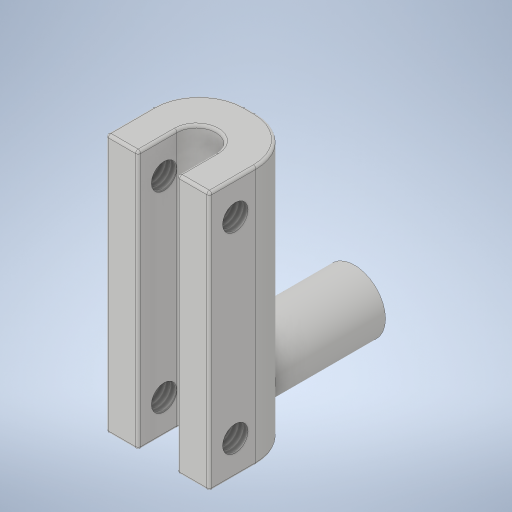
# Autodesk Inventor part: StepperToSpout_Gerion_V3
Saved by Autodesk Inventor 2023 (Build 270158000, 158)
## iProperties
Created: 2019-09-20
Part Number: StepperToSpout_Gerion_V3
Material: Generic
Document SubType Name: Modeling
Designer: Xiaonan Richard Sun
Density: 1 g/cm^3
Appearance: Default
Author: Xiaonan Richard Sun
Autodesk Inventor part; units mm, degrees
ref_plane "YZ Plane" through (0, 0, 0) normal (1, 0, 0) x (0, 1, 0)
ref_plane "XZ Plane" through (0, 0, 0) normal (0, 1, 0) x (-1, 0, 0)
ref_plane "XY Plane" through (0, 0, 0) normal (0, 0, 1) x (1, 0, 0)
sketch "Sketch1" plane through (0, 0, 0) normal (0, 0, 1) x (1, 0, 0)
  line L0 (0, 0) -> (10, 0)
  line L1 (10, 0) -> (10, 25)
  line L2 (10, 25) -> (0, 25)
  line L3 (0, 25) -> (0, 0)
  dimension "d0" = 10
  dimension "d1" = 25
  constraints: 8 end point, 2 parallel, 1 horizontal, 1 perpendicular
  measures "d0" distance of L2.end L1.end
  measures "d1" distance of L1.end L0.end
extrude "Extrusion1" add sketch "Sketch1" along normal blind 9
sketch "Sketch2" plane through (0, 0, 0) normal (0, 0, -1) x (-1, 0, 0)
  arc A0 (-3.4183, 2.63) -> (-6.5817, 2.63) centre (-5, 4) ccw
  arc A1 (-3.4183, 2.63) -> (-6.5817, 2.63) centre (-5, 4) ccw
  circle A2 centre (-5, 4) radius 3
  line L0 (0, 25) -> (0, 0) construction
  line L1 (0, 0) -> (-10, 0) construction
  line L2 (-6.5817, 2.63) -> (-3.4183, 2.63)
  line L3 (-5, 0) -> (-5, 25) construction
  line L4 (-10, 25) -> (0, 25) construction
  dimension "d7" = 4.185
  dimension "d9" = 6
  dimension "d35" = 3.1633
  dimension "d50" = 4
  constraints: 4 end point, 4 point on circle, 3 centre point, 2 midpoint, 1 coincident, 1 concentric, 1 horizontal, 1 point on line
  measures "d7" diameter of A0
  measures "d9" diameter of A2
  measures "d35" distance of L2.start L2.end
  measures "d50" distance from line of L1 A0.centre
extrude "Extrusion2" add sketch "Sketch2" along normal blind 10
sketch "Sketch4" plane through (0, 25, 0) normal (0, 1, 0) x (1, 0, 0)
  arc A0 (6.875, -5.25) -> (3.125, -5.25) centre (5, -5.25) ccw
  line L0 (3.125, -5.25) -> (3.125, -9)
  line L1 (6.875, -9) -> (6.875, -5.25)
  line L2 (10, -9) -> (0, -9) construction
  line L3 (6.875, -9) -> (3.125, -9)
  line L4 (10, 0) -> (0, 0) construction
  line L5 (5, 0) -> (5, -9) construction
  dimension "d14" = 3.75
  dimension "d39" = 3.75
  dimension "d53" = 3.75
  constraints: 8 end point, 3 point on line, 2 midpoint, 2 point on circle, 2 tangent, 1 centre point, 1 collinear, 1 perpendicular, 1 vertical
  measures "d14" diameter of A0
  measures "d39" distance between parallel lines of L0 L1
  measures "d53" distance from line of A0.centre L2
extrude "Extrusion4" cut sketch "Sketch4" against normal blind 25
sketch "Sketch8" plane through (0, 0, 9) normal (0, 0, 1) x (1, 0, 0)
  line L0 (2.3, 19) -> (7.7, 19)
  line L1 (7.7, 19) -> (7.7, 6)
  line L2 (7.7, 6) -> (2.3, 6)
  line L3 (2.3, 6) -> (2.3, 19)
  line L4 (6.875, 25) -> (6.875, 0) construction
  line L5 (6.875, 0) -> (10, 0) construction
  line L6 (10, 0) -> (10, 25) construction
  line L7 (10, 25) -> (6.875, 25) construction
  line L8 (3.125, 0) -> (3.125, 25) construction
  line L9 (3.125, 25) -> (0, 25) construction
  line L10 (0, 25) -> (0, 0) construction
  line L11 (0, 0) -> (3.125, 0) construction
  dimension "d54" = 6
  dimension "d55" = 6
  dimension "d56" = 2.3
  dimension "d57" = 2.3
  constraints: 8 end point, 2 parallel, 1 horizontal, 1 perpendicular
  measures "d54" distance between parallel lines of L5 L2
  measures "d55" distance between parallel lines of L7 L0
  measures "d56" distance between parallel lines of L6 L1
  measures "d57" distance between parallel lines of L10 L3
extrude "Extrusion6" [suppressed]
sketch "Sketch6" plane through (0, 6.7085, 2.6824) normal (-1, 0, 0) x (0, 0, 1)
  line L0 (-2.6824, 18.2915) -> (6.3176, 18.2915) construction
  line L1 (6.3176, 18.2915) -> (6.3176, -6.7085) construction
  line L2 (-2.6824, -6.7085) -> (6.3176, -6.7085) construction
  point P0 (3.8176, 15.0415)
  point P1 (3.8176, -3.4585)
  dimension "d47" = 3.25
  dimension "d58" = 2.5
  dimension "d59" = 3.25
  dimension "d60" = 2.5
  measures "d47" distance from line of point (3.818, 15.042) L0
  measures "d58" distance from line of L1 point (3.818, 15.042)
  measures "d59" distance from line of L2 point (3.818, -3.458)
  measures "d60" distance from line of L1 point (3.818, -3.458)
hole "Hole1" at (0, 21.75, 6.5) at (0, 3.25, 6.5) direction (1, 0, 0) diameter 2.459 end through all thread size "M3x0.5" class "6H" standard "ISO Metric profile"
fillet "Fillet2" radius 4.5 2 edges at (10, 12.5, 0) (0, 12.5, 0)
fillet "Fillet2" radius 0.25 21 edges at (10, 12.5, 9) (6.875, 12.5, 9) (3.125, 12.5, 9) (0, 12.5, 9) (1.5625, 25, 9) (1.5625, 0, 9) (5, 25, 3.375) (6.875, 25, 7.125) (3.125, 25, 7.125) (5, 0, 3.375) (6.875, 0, 7.125) (3.125, 0, 7.125) (8.4375, 25, 9) (8.4375, 0, 9) (10, 25, 4.5) (10, 0, 4.5) (5, 25, 0) (5, 0, 0) (0, 0, 4.5) (0, 25, 4.5) (8, 4, 0)
sketch "Sketch9" plane through (5, 4, -10) normal (0, 0, -1) x (-1, 0, 0)
  arc A0 (1.5817, -1.37) -> (-1.5817, -1.37) centre (0, 0) ccw construction
  arc A1 (0.4615, 2.9643) -> (-0.4615, 2.9643) centre (0, 0) ccw construction
  circle A2 centre (0, 0) radius 2.0925
  point P0 (5, -4)
  point P1 (-2.7692, 1.1538)
  point P2 (2.7692, 1.1538)
  constraints: 1 centre point, 1 coincident, 1 concentric
extrude "Extrusion7" cut sketch "Sketch9" against normal up to surface (10 mm away)
sketch "Sketch10" plane through (0, 0, 0) normal (0, 0, -1) x (-1, 0, 0)
  line L0 (-3, 16) -> (-3, 8) construction
  line L1 (-3, 8) -> (-7, 8) construction
  line L2 (-7, 8) -> (-7, 16) construction
  line L3 (-7, 16) -> (-3, 16) construction
  arc A0 (-4.5, 7.2113) -> (-5.5, 7.2113) centre (-5, 4) ccw construction
  line L4 (-5, 7.25) -> (-5, 25) construction
  line L5 (-4.5, 25) -> (-5.5, 25) construction
  line L6 (-3.5491, 14.0041) -> (-4.5491, 14.3485)
  line L7 (-4.5491, 14.3485) -> (-4.5491, 14.4919)
  line L8 (-4.5491, 14.4919) -> (-3.5491, 14.8363)
  line L9 (-3.5491, 14.8363) -> (-3.5491, 14.6937)
  line L10 (-3.5491, 14.6937) -> (-4.3798, 14.4165)
  line L11 (-4.3798, 14.4165) -> (-3.5491, 14.1394)
  line L12 (-3.5491, 14.1394) -> (-3.5491, 14.0041)
  spline S0 degree 2 poles (-4.5661, 13.5924) (-4.5661, 13.7723) (-4.3644, 13.97) (-4.178, 13.97) knots 0 0 0 1 2 2 2
  spline S1 degree 2 poles (-4.178, 13.97) (-3.9948, 13.97) (-3.7777, 13.778) (-3.7777, 13.6232) knots 0 0 0 1 2 2 2
  spline S2 degree 2 poles (-3.7777, 13.6232) (-3.7777, 13.5535) (-3.8182, 13.4457) (-3.8611, 13.406) knots 0 0 0 1 2 2 2
  spline S3 degree 2 poles (-3.8611, 13.406) (-3.9041, 13.3655) (-4.0281, 13.3225) (-4.118, 13.3225) knots 0 0 0 1 2 2 2
  line L13 (-4.118, 13.3225) -> (-4.1869, 13.3225)
  line L14 (-4.1869, 13.3225) -> (-4.1869, 13.842)
  spline S4 degree 2 poles (-4.1869, 13.842) (-4.3174, 13.842) (-4.4559, 13.7107) (-4.4559, 13.594) knots 0 0 0 1 2 2 2
  spline S5 degree 2 poles (-4.4559, 13.594) (-4.4559, 13.5527) (-4.4373, 13.4724) (-4.4227, 13.44) knots 0 0 0 1 2 2 2
  spline S6 degree 2 poles (-4.4227, 13.44) (-4.4065, 13.406) (-4.3781, 13.359) (-4.3652, 13.3436) knots 0 0 0 1 2 2 2
  line L15 (-4.3652, 13.3436) -> (-4.3652, 13.3363)
  line L16 (-4.3652, 13.3363) -> (-4.5029, 13.3363)
  spline S7 degree 2 poles (-4.5029, 13.3363) (-4.5119, 13.3582) (-4.5378, 13.4246) (-4.5451, 13.4506) knots 0 0 0 1 2 2 2
  spline S8 degree 2 poles (-4.5451, 13.4506) (-4.5556, 13.487) (-4.5661, 13.547) (-4.5661, 13.5924) knots 0 0 0 1 2 2 2
  spline S9 degree 2 poles (-4.0905, 13.4457) (-4.0394, 13.4473) (-3.9649, 13.4684) (-3.9397, 13.4887) knots 0 0 0 1 2 2 2
  spline S10 degree 2 poles (-3.9397, 13.4887) (-3.9114, 13.5105) (-3.8814, 13.5794) (-3.8814, 13.6305) knots 0 0 0 1 2 2 2
  spline S11 degree 2 poles (-3.8814, 13.6305) (-3.8814, 13.6807) (-3.9114, 13.7512) (-3.9405, 13.7804) knots 0 0 0 1 2 2 2
  spline S12 degree 2 poles (-3.9405, 13.7804) (-3.9705, 13.8088) (-4.0426, 13.8379) (-4.0905, 13.842) knots 0 0 0 1 2 2 2
  line L17 (-4.0905, 13.842) -> (-4.0905, 13.4457)
  line L18 (-3.9341, 12.7966) -> (-3.9341, 12.8031)
  spline S13 degree 2 poles (-3.9341, 12.8031) (-3.93, 12.8177) (-3.9284, 12.8493) (-3.9284, 12.8712) knots 0 0 0 1 2 2 2
  spline S14 degree 2 poles (-3.9284, 12.8712) (-3.9284, 12.9222) (-3.973, 13.0227) (-4.0167, 13.0681) knots 0 0 0 1 2 2 2
  line L19 (-4.0167, 13.0681) -> (-4.5491, 13.0681)
  line L20 (-4.5491, 13.0681) -> (-4.5491, 13.1945)
  line L21 (-4.5491, 13.1945) -> (-3.7987, 13.1945)
  line L22 (-3.7987, 13.1945) -> (-3.7987, 13.0681)
  line L23 (-3.7987, 13.0681) -> (-3.9106, 13.0681)
  spline S15 degree 2 poles (-3.9106, 13.0681) (-3.849, 12.9992) (-3.7987, 12.8963) (-3.7987, 12.8477) knots 0 0 0 1 2 2 2
  spline S16 degree 2 poles (-3.7987, 12.8477) (-3.7987, 12.8282) (-3.8003, 12.8088) (-3.8028, 12.7966) knots 0 0 0 1 2 2 2
  line L24 (-3.8028, 12.7966) -> (-3.9341, 12.7966)
  spline S17 degree 2 poles (-4.567, 12.4959) (-4.567, 12.5713) (-4.5264, 12.7018) (-4.5037, 12.7447) knots 0 0 0 1 2 2 2
  line L25 (-4.5037, 12.7447) -> (-4.3619, 12.7447)
  line L26 (-4.3619, 12.7447) -> (-4.3619, 12.7382)
  spline S18 degree 2 poles (-4.3619, 12.7382) (-4.3749, 12.722) (-4.4057, 12.6783) (-4.4227, 12.6418) knots 0 0 0 1 2 2 2
  spline S19 degree 2 poles (-4.4227, 12.6418) (-4.4381, 12.6102) (-4.4608, 12.5324) (-4.4608, 12.4911) knots 0 0 0 1 2 2 2
  spline S20 degree 2 poles (-4.4608, 12.4911) (-4.4608, 12.4611) (-4.447, 12.3922) (-4.4357, 12.376) knots 0 0 0 1 2 2 2
  spline S21 degree 2 poles (-4.4357, 12.376) (-4.4203, 12.3525) (-4.3854, 12.3314) (-4.3498, 12.3314) knots 0 0 0 1 2 2 2
  spline S22 degree 2 poles (-4.3498, 12.3314) (-4.3052, 12.3314) (-4.259, 12.3801) (-4.2436, 12.4425) knots 0 0 0 1 2 2 2
  spline S23 degree 2 poles (-4.2436, 12.4425) (-4.2379, 12.4668) (-4.2217, 12.5446) (-4.2128, 12.5778) knots 0 0 0 1 2 2 2
  spline S24 degree 2 poles (-4.2128, 12.5778) (-4.1877, 12.6637) (-4.084, 12.7415) (-4.0102, 12.7415) knots 0 0 0 1 2 2 2
  spline S25 degree 2 poles (-4.0102, 12.7415) (-3.9081, 12.7415) (-3.7809, 12.5883) (-3.7809, 12.4619) knots 0 0 0 1 2 2 2
  spline S26 degree 2 poles (-3.7809, 12.4619) (-3.7809, 12.3995) (-3.8117, 12.2731) (-3.8352, 12.2301) knots 0 0 0 1 2 2 2
  line L27 (-3.8352, 12.2301) -> (-3.9705, 12.2301)
  line L28 (-3.9705, 12.2301) -> (-3.9705, 12.2366)
  spline S27 degree 2 poles (-3.9705, 12.2366) (-3.9316, 12.2853) (-3.8871, 12.4036) (-3.8871, 12.4643) knots 0 0 0 1 2 2 2
  spline S28 degree 2 poles (-3.8871, 12.4643) (-3.8871, 12.5267) (-3.9397, 12.6126) (-3.9924, 12.6126) knots 0 0 0 1 2 2 2
  spline S29 degree 2 poles (-3.9924, 12.6126) (-4.0402, 12.6126) (-4.0864, 12.5616) (-4.101, 12.5049) knots 0 0 0 1 2 2 2
  spline S30 degree 2 poles (-4.101, 12.5049) (-4.1083, 12.4773) (-4.1229, 12.4076) (-4.1318, 12.3695) knots 0 0 0 1 2 2 2
  spline S31 degree 2 poles (-4.1318, 12.3695) (-4.1529, 12.2869) (-4.2493, 12.2026) (-4.3328, 12.2026) knots 0 0 0 1 2 2 2
  spline S32 degree 2 poles (-4.3328, 12.2026) (-4.3814, 12.2026) (-4.4673, 12.2407) (-4.4989, 12.278) knots 0 0 0 1 2 2 2
  spline S33 degree 2 poles (-4.4989, 12.278) (-4.5321, 12.3177) (-4.567, 12.419) (-4.567, 12.4959) knots 0 0 0 1 2 2 2
  line L29 (-4.5491, 11.9562) -> (-4.5491, 12.0827)
  line L30 (-4.5491, 12.0827) -> (-3.7987, 12.0827)
  line L31 (-3.7987, 12.0827) -> (-3.7987, 11.9562)
  line L32 (-3.7987, 11.9562) -> (-4.5491, 11.9562)
  line L33 (-3.6739, 11.9473) -> (-3.6739, 12.0908)
  line L34 (-3.6739, 12.0908) -> (-3.5426, 12.0908)
  line L35 (-3.5426, 12.0908) -> (-3.5426, 11.9473)
  line L36 (-3.5426, 11.9473) -> (-3.6739, 11.9473)
  spline S34 degree 2 poles (-4.1739, 11.154) (-4.3636, 11.154) (-4.5702, 11.3363) (-4.5702, 11.4887) knots 0 0 0 1 2 2 2
  spline S35 degree 2 poles (-4.5702, 11.4887) (-4.5702, 11.6451) (-4.3571, 11.8241) (-4.1739, 11.8241) knots 0 0 0 1 2 2 2
  spline S36 degree 2 poles (-4.1739, 11.8241) (-3.9859, 11.8241) (-3.7777, 11.6394) (-3.7777, 11.4887) knots 0 0 0 1 2 2 2
  spline S37 degree 2 poles (-3.7777, 11.4887) (-3.7777, 11.3363) (-3.9851, 11.154) (-4.1739, 11.154) knots 0 0 0 1 2 2 2
  spline S38 degree 2 poles (-4.1739, 11.2844) (-4.0281, 11.2844) (-3.8862, 11.3906) (-3.8862, 11.4887) knots 0 0 0 1 2 2 2
  spline S39 degree 2 poles (-3.8862, 11.4887) (-3.8862, 11.5867) (-4.0281, 11.6937) (-4.1739, 11.6937) knots 0 0 0 1 2 2 2
  spline S40 degree 2 poles (-4.1739, 11.6937) (-4.3157, 11.6937) (-4.4616, 11.5867) (-4.4616, 11.4887) knots 0 0 0 1 2 2 2
  spline S41 degree 2 poles (-4.4616, 11.4887) (-4.4616, 11.3914) (-4.3182, 11.2844) (-4.1739, 11.2844) knots 0 0 0 1 2 2 2
  line L37 (-4.5491, 10.4352) -> (-4.5491, 10.5616)
  line L38 (-4.5491, 10.5616) -> (-4.1213, 10.5616)
  spline S42 degree 2 poles (-4.1213, 10.5616) (-4.0694, 10.5616) (-3.9802, 10.5713) (-3.9535, 10.5859) knots 0 0 0 1 2 2 2
  spline S43 degree 2 poles (-3.9535, 10.5859) (-3.9251, 10.6013) (-3.8976, 10.6564) (-3.8976, 10.7034) knots 0 0 0 1 2 2 2
  spline S44 degree 2 poles (-3.8976, 10.7034) (-3.8976, 10.7504) (-3.9478, 10.8501) (-3.9884, 10.8979) knots 0 0 0 1 2 2 2
  line L39 (-3.9884, 10.8979) -> (-4.5491, 10.8979)
  line L40 (-4.5491, 10.8979) -> (-4.5491, 11.0243)
  line L41 (-4.5491, 11.0243) -> (-3.7987, 11.0243)
  line L42 (-3.7987, 11.0243) -> (-3.7987, 10.8979)
  line L43 (-3.7987, 10.8979) -> (-3.8822, 10.8979)
  spline S45 degree 2 poles (-3.8822, 10.8979) (-3.8311, 10.8412) (-3.7777, 10.7318) (-3.7777, 10.6702) knots 0 0 0 1 2 2 2
  spline S46 degree 2 poles (-3.7777, 10.6702) (-3.7777, 10.56) (-3.9235, 10.4352) (-4.0621, 10.4352) knots 0 0 0 1 2 2 2
  line L44 (-4.0621, 10.4352) -> (-4.5491, 10.4352)
  spline S47 degree 2 poles (-3.6439, 9.577) (-3.6439, 9.6135) (-3.6618, 9.6856) (-3.6755, 9.7204) knots 0 0 0 1 2 2 2
  spline S48 degree 2 poles (-3.6755, 9.7204) (-3.6893, 9.7528) (-3.7185, 9.8006) (-3.7315, 9.8193) knots 0 0 0 1 2 2 2
  line L45 (-3.7315, 9.8193) -> (-3.7315, 9.8274)
  line L46 (-3.7315, 9.8274) -> (-3.5896, 9.8274)
  spline S49 degree 2 poles (-3.5896, 9.8274) (-3.5661, 9.7836) (-3.5281, 9.6337) (-3.5281, 9.5665) knots 0 0 0 1 2 2 2
  spline S50 degree 2 poles (-3.5281, 9.5665) (-3.5281, 9.4984) (-3.5556, 9.3971) (-3.5848, 9.3558) knots 0 0 0 1 2 2 2
  spline S51 degree 2 poles (-3.5848, 9.3558) (-3.6164, 9.312) (-3.708, 9.2666) (-3.7696, 9.2666) knots 0 0 0 1 2 2 2
  spline S52 degree 2 poles (-3.7696, 9.2666) (-3.8522, 9.2666) (-3.977, 9.3752) (-3.9932, 9.4514) knots 0 0 0 1 2 2 2
  line L47 (-3.9932, 9.4514) -> (-4.0029, 9.4514)
  spline S53 degree 2 poles (-4.0029, 9.4514) (-4.0094, 9.4198) (-4.0386, 9.3477) (-4.0678, 9.3169) knots 0 0 0 1 2 2 2
  spline S54 degree 2 poles (-4.0678, 9.3169) (-4.0961, 9.2861) (-4.1869, 9.2472) (-4.2525, 9.2472) knots 0 0 0 1 2 2 2
  spline S55 degree 2 poles (-4.2525, 9.2472) (-4.3198, 9.2472) (-4.4341, 9.2934) (-4.4778, 9.3355) knots 0 0 0 1 2 2 2
  spline S56 degree 2 poles (-4.4778, 9.3355) (-4.5232, 9.3793) (-4.5702, 9.5032) (-4.5702, 9.5818) knots 0 0 0 1 2 2 2
  spline S57 degree 2 poles (-4.5702, 9.5818) (-4.5702, 9.6572) (-4.5337, 9.8047) (-4.5086, 9.8549) knots 0 0 0 1 2 2 2
  line L48 (-4.5086, 9.8549) -> (-4.3668, 9.8549)
  line L49 (-4.3668, 9.8549) -> (-4.3668, 9.8452)
  spline S58 degree 2 poles (-4.3668, 9.8452) (-4.3976, 9.8031) (-4.4543, 9.6605) (-4.4543, 9.59) knots 0 0 0 1 2 2 2
  spline S59 degree 2 poles (-4.4543, 9.59) (-4.4543, 9.5486) (-4.4284, 9.466) (-4.3984, 9.4384) knots 0 0 0 1 2 2 2
  spline S60 degree 2 poles (-4.3984, 9.4384) (-4.3684, 9.4117) (-4.2971, 9.3833) (-4.2428, 9.3833) knots 0 0 0 1 2 2 2
  spline S61 degree 2 poles (-4.2428, 9.3833) (-4.1885, 9.3833) (-4.118, 9.4149) (-4.0978, 9.4433) knots 0 0 0 1 2 2 2
  spline S62 degree 2 poles (-4.0978, 9.4433) (-4.0775, 9.4716) (-4.0621, 9.5486) (-4.0621, 9.594) knots 0 0 0 1 2 2 2
  line L50 (-4.0621, 9.594) -> (-4.0621, 9.6507)
  line L51 (-4.0621, 9.6507) -> (-3.9511, 9.6507)
  line L52 (-3.9511, 9.6507) -> (-3.9511, 9.6062)
  spline S63 degree 2 poles (-3.9511, 9.6062) (-3.9511, 9.5162) (-3.8652, 9.4028) (-3.7833, 9.4028) knots 0 0 0 1 2 2 2
  spline S64 degree 2 poles (-3.7833, 9.4028) (-3.7452, 9.4028) (-3.6909, 9.4319) (-3.6747, 9.4554) knots 0 0 0 1 2 2 2
  spline S65 degree 2 poles (-3.6747, 9.4554) (-3.6577, 9.4806) (-3.6439, 9.5421) (-3.6439, 9.577) knots 0 0 0 1 2 2 2
  spline S66 degree 2 poles (-5.8885, 14.1653) (-5.963, 14.1653) (-6.0773, 14.222) (-6.1146, 14.269) knots 0 0 0 1 2 2 2
  spline S67 degree 2 poles (-6.1146, 14.269) (-6.1583, 14.3258) (-6.1956, 14.4546) (-6.1956, 14.5567) knots 0 0 0 1 2 2 2
  line L53 (-6.1956, 14.5567) -> (-6.1956, 14.8436)
  line L54 (-6.1956, 14.8436) -> (-5.1956, 14.8436)
  line L55 (-5.1956, 14.8436) -> (-5.1956, 14.5786)
  spline S68 degree 2 poles (-5.1956, 14.5786) (-5.1956, 14.4716) (-5.2094, 14.3647) (-5.2361, 14.316) knots 0 0 0 1 2 2 2
  spline S69 degree 2 poles (-5.2361, 14.316) (-5.2645, 14.2618) (-5.3577, 14.2123) (-5.4209, 14.2123) knots 0 0 0 1 2 2 2
  spline S70 degree 2 poles (-5.4209, 14.2123) (-5.4914, 14.2123) (-5.6032, 14.2869) (-5.6348, 14.3525) knots 0 0 0 1 2 2 2
  line L56 (-5.6348, 14.3525) -> (-5.6397, 14.3525)
  spline S71 degree 2 poles (-5.6397, 14.3525) (-5.664, 14.2634) (-5.7928, 14.1653) (-5.8885, 14.1653) knots 0 0 0 1 2 2 2
  spline S72 degree 2 poles (-5.8941, 14.3039) (-5.8374, 14.3039) (-5.7645, 14.3363) (-5.7386, 14.3849) knots 0 0 0 1 2 2 2
  spline S73 degree 2 poles (-5.7386, 14.3849) (-5.7223, 14.4165) (-5.7126, 14.4911) (-5.7126, 14.56) knots 0 0 0 1 2 2 2
  line L57 (-5.7126, 14.56) -> (-5.7126, 14.7107)
  line L58 (-5.7126, 14.7107) -> (-6.0822, 14.7107)
  line L59 (-6.0822, 14.7107) -> (-6.0822, 14.6029)
  spline S74 degree 2 poles (-6.0822, 14.6029) (-6.0822, 14.5154) (-6.0659, 14.4149) (-6.04, 14.376) knots 0 0 0 1 2 2 2
  spline S75 degree 2 poles (-6.04, 14.376) (-6.0133, 14.3387) (-5.9468, 14.3039) (-5.8941, 14.3039) knots 0 0 0 1 2 2 2
  spline S76 degree 2 poles (-5.4395, 14.3509) (-5.4039, 14.3509) (-5.3504, 14.3752) (-5.335, 14.4019) knots 0 0 0 1 2 2 2
  spline S77 degree 2 poles (-5.335, 14.4019) (-5.3172, 14.4344) (-5.3091, 14.513) (-5.3091, 14.5835) knots 0 0 0 1 2 2 2
  line L60 (-5.3091, 14.5835) -> (-5.3091, 14.7107)
  line L61 (-5.3091, 14.7107) -> (-5.6016, 14.7107)
  line L62 (-5.6016, 14.7107) -> (-5.6016, 14.56)
  spline S78 degree 2 poles (-5.6016, 14.56) (-5.6016, 14.4976) (-5.5886, 14.4384) (-5.5684, 14.4068) knots 0 0 0 1 2 2 2
  spline S79 degree 2 poles (-5.5684, 14.4068) (-5.5489, 14.376) (-5.4865, 14.3509) (-5.4395, 14.3509) knots 0 0 0 1 2 2 2
  line L63 (-5.4452, 13.4538) -> (-6.4719, 13.8574)
  line L64 (-6.4719, 13.8574) -> (-6.4719, 13.9927)
  line L65 (-6.4719, 13.9927) -> (-6.1591, 13.8582)
  line L66 (-6.1591, 13.8582) -> (-5.4452, 14.1305)
  line L67 (-5.4452, 14.1305) -> (-5.4452, 13.9943)
  line L68 (-5.4452, 13.9943) -> (-6.0011, 13.7893)
  line L69 (-6.0011, 13.7893) -> (-5.4452, 13.5851)
  line L70 (-5.4452, 13.5851) -> (-5.4452, 13.4538)
  spline S80 degree 2 poles (-6.2151, 12.5) (-6.2151, 12.6062) (-6.1502, 12.782) (-6.0846, 12.8452) knots 0 0 0 1 2 2 2
  spline S81 degree 2 poles (-6.0846, 12.8452) (-6.0181, 12.9084) (-5.822, 12.9757) (-5.6948, 12.9757) knots 0 0 0 1 2 2 2
  spline S82 degree 2 poles (-5.6948, 12.9757) (-5.574, 12.9757) (-5.3828, 12.9076) (-5.3147, 12.8444) knots 0 0 0 1 2 2 2
  spline S83 degree 2 poles (-5.3147, 12.8444) (-5.2491, 12.7836) (-5.1778, 12.6053) (-5.1778, 12.4992) knots 0 0 0 1 2 2 2
  spline S84 degree 2 poles (-5.1778, 12.4992) (-5.1778, 12.4481) (-5.1924, 12.3558) (-5.2053, 12.3136) knots 0 0 0 1 2 2 2
  spline S85 degree 2 poles (-5.2053, 12.3136) (-5.2151, 12.2796) (-5.2507, 12.1969) (-5.2637, 12.1718) knots 0 0 0 1 2 2 2
  line L71 (-5.2637, 12.1718) -> (-5.4241, 12.1718)
  line L72 (-5.4241, 12.1718) -> (-5.4241, 12.1831)
  spline S86 degree 2 poles (-5.4241, 12.1831) (-5.4022, 12.2083) (-5.3625, 12.2609) (-5.3398, 12.3096) knots 0 0 0 1 2 2 2
  spline S87 degree 2 poles (-5.3398, 12.3096) (-5.3196, 12.3501) (-5.2928, 12.4546) (-5.2928, 12.5146) knots 0 0 0 1 2 2 2
  spline S88 degree 2 poles (-5.2928, 12.5146) (-5.2928, 12.6588) (-5.51, 12.8371) (-5.6907, 12.8371) knots 0 0 0 1 2 2 2
  spline S89 degree 2 poles (-5.6907, 12.8371) (-5.7912, 12.8371) (-5.942, 12.7901) (-5.9938, 12.7455) knots 0 0 0 1 2 2 2
  spline S90 degree 2 poles (-5.9938, 12.7455) (-6.0457, 12.7026) (-6.1, 12.581) (-6.1, 12.5049) knots 0 0 0 1 2 2 2
  spline S91 degree 2 poles (-6.1, 12.5049) (-6.1, 12.4489) (-6.0838, 12.3371) (-6.0676, 12.299) knots 0 0 0 1 2 2 2
  line L73 (-6.0676, 12.299) -> (-5.8091, 12.299)
  line L74 (-5.8091, 12.299) -> (-5.8091, 12.5308)
  line L75 (-5.8091, 12.5308) -> (-5.6924, 12.5308)
  line L76 (-5.6924, 12.5308) -> (-5.6924, 12.1677)
  line L77 (-5.6924, 12.1677) -> (-6.1292, 12.1677)
  spline S92 degree 2 poles (-6.1292, 12.1677) (-6.1405, 12.1929) (-6.1753, 12.2788) (-6.1859, 12.3152) knots 0 0 0 1 2 2 2
  spline S93 degree 2 poles (-6.1859, 12.3152) (-6.2005, 12.3647) (-6.2151, 12.4441) (-6.2151, 12.5) knots 0 0 0 1 2 2 2
  spline S94 degree 2 poles (-6.2126, 11.6848) (-6.2126, 11.8647) (-6.0108, 12.0624) (-5.8245, 12.0624) knots 0 0 0 1 2 2 2
  spline S95 degree 2 poles (-5.8245, 12.0624) (-5.6413, 12.0624) (-5.4241, 11.8703) (-5.4241, 11.7156) knots 0 0 0 1 2 2 2
  spline S96 degree 2 poles (-5.4241, 11.7156) (-5.4241, 11.6459) (-5.4646, 11.5381) (-5.5076, 11.4984) knots 0 0 0 1 2 2 2
  spline S97 degree 2 poles (-5.5076, 11.4984) (-5.5505, 11.4579) (-5.6745, 11.4149) (-5.7645, 11.4149) knots 0 0 0 1 2 2 2
  line L78 (-5.7645, 11.4149) -> (-5.8334, 11.4149)
  line L79 (-5.8334, 11.4149) -> (-5.8334, 11.9344)
  spline S98 degree 2 poles (-5.8334, 11.9344) (-5.9638, 11.9344) (-6.1024, 11.8031) (-6.1024, 11.6864) knots 0 0 0 1 2 2 2
  spline S99 degree 2 poles (-6.1024, 11.6864) (-6.1024, 11.6451) (-6.0838, 11.5648) (-6.0692, 11.5324) knots 0 0 0 1 2 2 2
  spline S100 degree 2 poles (-6.0692, 11.5324) (-6.053, 11.4984) (-6.0246, 11.4514) (-6.0116, 11.436) knots 0 0 0 1 2 2 2
  line L80 (-6.0116, 11.436) -> (-6.0116, 11.4287)
  line L81 (-6.0116, 11.4287) -> (-6.1494, 11.4287)
  spline S101 degree 2 poles (-6.1494, 11.4287) (-6.1583, 11.4506) (-6.1843, 11.517) (-6.1916, 11.5429) knots 0 0 0 1 2 2 2
  spline S102 degree 2 poles (-6.1916, 11.5429) (-6.2021, 11.5794) (-6.2126, 11.6394) (-6.2126, 11.6848) knots 0 0 0 1 2 2 2
  spline S103 degree 2 poles (-5.7369, 11.5381) (-5.6859, 11.5397) (-5.6113, 11.5608) (-5.5862, 11.581) knots 0 0 0 1 2 2 2
  spline S104 degree 2 poles (-5.5862, 11.581) (-5.5578, 11.6029) (-5.5279, 11.6718) (-5.5279, 11.7229) knots 0 0 0 1 2 2 2
  spline S105 degree 2 poles (-5.5279, 11.7229) (-5.5279, 11.7731) (-5.5578, 11.8436) (-5.587, 11.8728) knots 0 0 0 1 2 2 2
  spline S106 degree 2 poles (-5.587, 11.8728) (-5.617, 11.9011) (-5.6891, 11.9303) (-5.7369, 11.9344) knots 0 0 0 1 2 2 2
  line L82 (-5.7369, 11.9344) -> (-5.7369, 11.5381)
  line L83 (-5.5805, 10.889) -> (-5.5805, 10.8955)
  spline S107 degree 2 poles (-5.5805, 10.8955) (-5.5765, 10.91) (-5.5749, 10.9417) (-5.5749, 10.9635) knots 0 0 0 1 2 2 2
  spline S108 degree 2 poles (-5.5749, 10.9635) (-5.5749, 11.0146) (-5.6194, 11.1151) (-5.6632, 11.1605) knots 0 0 0 1 2 2 2
  line L84 (-5.6632, 11.1605) -> (-6.1956, 11.1605)
  line L85 (-6.1956, 11.1605) -> (-6.1956, 11.2869)
  line L86 (-6.1956, 11.2869) -> (-5.4452, 11.2869)
  line L87 (-5.4452, 11.2869) -> (-5.4452, 11.1605)
  line L88 (-5.4452, 11.1605) -> (-5.557, 11.1605)
  spline S109 degree 2 poles (-5.557, 11.1605) (-5.4954, 11.0916) (-5.4452, 10.9887) (-5.4452, 10.94) knots 0 0 0 1 2 2 2
  spline S110 degree 2 poles (-5.4452, 10.94) (-5.4452, 10.9206) (-5.4468, 10.9011) (-5.4492, 10.889) knots 0 0 0 1 2 2 2
  line L89 (-5.4492, 10.889) -> (-5.5805, 10.889)
  line L90 (-6.1956, 10.6621) -> (-6.1956, 10.7885)
  line L91 (-6.1956, 10.7885) -> (-5.4452, 10.7885)
  line L92 (-5.4452, 10.7885) -> (-5.4452, 10.6621)
  line L93 (-5.4452, 10.6621) -> (-6.1956, 10.6621)
  line L94 (-5.3204, 10.6532) -> (-5.3204, 10.7966)
  line L95 (-5.3204, 10.7966) -> (-5.1891, 10.7966)
  line L96 (-5.1891, 10.7966) -> (-5.1891, 10.6532)
  line L97 (-5.1891, 10.6532) -> (-5.3204, 10.6532)
  spline S111 degree 2 poles (-5.8204, 9.8598) (-6.01, 9.8598) (-6.2167, 10.0421) (-6.2167, 10.1945) knots 0 0 0 1 2 2 2
  spline S112 degree 2 poles (-6.2167, 10.1945) (-6.2167, 10.3509) (-6.0035, 10.53) (-5.8204, 10.53) knots 0 0 0 1 2 2 2
  spline S113 degree 2 poles (-5.8204, 10.53) (-5.6324, 10.53) (-5.4241, 10.3452) (-5.4241, 10.1945) knots 0 0 0 1 2 2 2
  spline S114 degree 2 poles (-5.4241, 10.1945) (-5.4241, 10.0421) (-5.6316, 9.8598) (-5.8204, 9.8598) knots 0 0 0 1 2 2 2
  spline S115 degree 2 poles (-5.8204, 9.9903) (-5.6745, 9.9903) (-5.5327, 10.0964) (-5.5327, 10.1945) knots 0 0 0 1 2 2 2
  spline S116 degree 2 poles (-5.5327, 10.1945) (-5.5327, 10.2925) (-5.6745, 10.3995) (-5.8204, 10.3995) knots 0 0 0 1 2 2 2
  spline S117 degree 2 poles (-5.8204, 10.3995) (-5.9622, 10.3995) (-6.1081, 10.2925) (-6.1081, 10.1945) knots 0 0 0 1 2 2 2
  spline S118 degree 2 poles (-6.1081, 10.1945) (-6.1081, 10.0972) (-5.9646, 9.9903) (-5.8204, 9.9903) knots 0 0 0 1 2 2 2
  line L98 (-6.1956, 9.141) -> (-6.1956, 9.2674)
  line L99 (-6.1956, 9.2674) -> (-5.7677, 9.2674)
  spline S119 degree 2 poles (-5.7677, 9.2674) (-5.7159, 9.2674) (-5.6267, 9.2771) (-5.6, 9.2917) knots 0 0 0 1 2 2 2
  spline S120 degree 2 poles (-5.6, 9.2917) (-5.5716, 9.3071) (-5.5441, 9.3622) (-5.5441, 9.4092) knots 0 0 0 1 2 2 2
  spline S121 degree 2 poles (-5.5441, 9.4092) (-5.5441, 9.4562) (-5.5943, 9.5559) (-5.6348, 9.6037) knots 0 0 0 1 2 2 2
  line L100 (-5.6348, 9.6037) -> (-6.1956, 9.6037)
  line L101 (-6.1956, 9.6037) -> (-6.1956, 9.7301)
  line L102 (-6.1956, 9.7301) -> (-5.4452, 9.7301)
  line L103 (-5.4452, 9.7301) -> (-5.4452, 9.6037)
  line L104 (-5.4452, 9.6037) -> (-5.5287, 9.6037)
  spline S122 degree 2 poles (-5.5287, 9.6037) (-5.4776, 9.547) (-5.4241, 9.4376) (-5.4241, 9.376) knots 0 0 0 1 2 2 2
  spline S123 degree 2 poles (-5.4241, 9.376) (-5.4241, 9.2658) (-5.57, 9.141) (-5.7086, 9.141) knots 0 0 0 1 2 2 2
  line L105 (-5.7086, 9.141) -> (-6.1956, 9.141)
  point P0 (0, 0)
  point P1 (-5, 8)
  dimension "d67" = 0.75
  dimension "d68" = 8
  dimension "d69" = 4
  constraints: 2 end point, 2 midpoint, 1 point on circle, 1 point on line, 2 other
  measures "d67" distance from line of L4.start L1
  measures "d68" distance of L0.start L0.end
  measures "d69" distance of L2.end L0.start
extrude "Extrusion8" cut sketch "Sketch10" against normal blind 0.15
body "Solid1"
